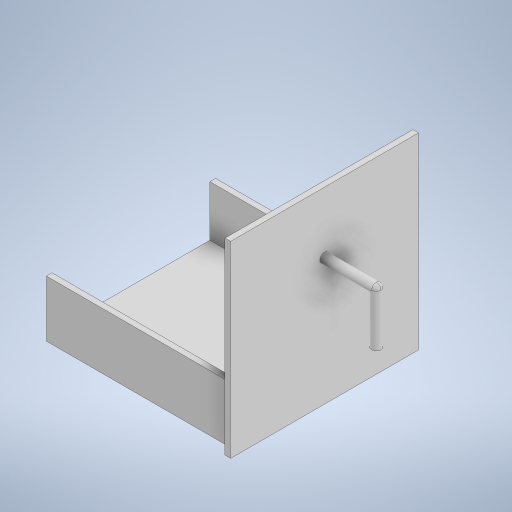
# Autodesk Inventor part: RS2_AshBucket
Saved by Autodesk Inventor 2024.3 (Build 283343000, 343)
## iProperties
Created: 2025-04-11
Part Number: RS2_AshBucket
Material: Generic
Document SubType Name: Modeling
Designer: ajclo
Density: 1 g/cm^3
Appearance: Default
Author: ajclo
Autodesk Inventor part; units mm, degrees
ref_plane "YZ Plane" through (0, 0, 0) normal (1, 0, 0) x (0, 1, 0)
ref_plane "XZ Plane" through (0, 0, 0) normal (0, 1, 0) x (-1, 0, 0)
ref_plane "XY Plane" through (0, 0, 0) normal (0, 0, 1) x (1, 0, 0)
sketch "Sketch1" plane through (0, 0, 0) normal (1, 0, 0) x (0, 1, 0)
  line L0 (0, 45) -> (30, 45)
  line L1 (30, 45) -> (30, -45)
  line L2 (30, -45) -> (0, -45)
  line L3 (0, -45) -> (0, 45)
  line L4 (30, 42) -> (3, 42)
  line L5 (3, 42) -> (3, -42)
  line L6 (3, -42) -> (30, -42)
  line L7 (30, -42) -> (30, 42)
  point P0 (0, 0)
  point P1 (30, -42)
  dimension "d0" = 45
  dimension "d1" = 90
  dimension "d2" = 30
  dimension "d3" = 0
  dimension "d4" = 3
  dimension "d5" = 3
  dimension "d6" = 3
  constraints: 16 end point, 4 parallel, 2 horizontal, 2 perpendicular, 1 point on line
  measures "d0" distance from line of L0 point (0, 0)
  measures "d1" distance of L0.end L1.end
  measures "d2" distance of L0.start L0.end
  measures "d3" distance from line of point (0, 0) L3
  measures "d4" distance between parallel lines of L2 L6
  measures "d5" distance between parallel lines of L3 L5
  measures "d6" distance between parallel lines of L0 L4
extrude "Extrusion1" add sketch "Sketch1" along normal blind 100 contours L0 L1 L4 L5 L6 L2 L3
sketch "Sketch2" plane through (100, 0, 0) normal (1, 0, 0) x (0, 0, -1)
  line L0 (-50, 0) -> (50, 0)
  line L1 (50, 0) -> (50, 100)
  line L2 (50, 100) -> (-50, 100)
  line L3 (-50, 100) -> (-50, 0)
  line L4 (-45, 0) -> (45, 0) projected
  point P0 (0, 0)
  point P1 (0, 0)
  dimension "d9" = 100
  dimension "d10" = 100
  constraints: 8 end point, 2 midpoint, 2 parallel, 1 horizontal, 1 perpendicular
  measures "d9" distance of L1.end L2.end
  measures "d10" distance of L0.end L1.end
extrude "Extrusion2" add sketch "Sketch2" along normal blind 3
sketch "Sketch4" plane through (0, 0, 0) normal (0, 0, 1) x (1, 0, 0)
  line L0 (103, 100) -> (103, 0) projected
  line L1 (103, 70) -> (133, 70)
  line L2 (133, 70) -> (133, 40)
  line L3 (133, 40) -> (128, 40)
  line L4 (128, 40) -> (128, 65)
  line L5 (128, 65) -> (103, 65)
  line L6 (100, 100) -> (103, 100) projected
  point P0 (0, 0)
  point P1 (115.5, 65)
  point P2 (118, 70)
  point P3 (128, 52.5)
  point P4 (101.5, 100)
  dimension "d13" = 5
  dimension "d14" = 5
  dimension "d15" = 30
  dimension "d16" = 30
  dimension "d17" = 30
  constraints: 10 end point, 4 midpoint, 4 perpendicular, 2 point on line, 1 horizontal
  measures "d13" vertical distance of point (115.5, 65) point (118, 70)
  measures "d14" distance from line of L2 point (128, 52.5)
  measures "d15" distance of L1.start L1.end
  measures "d16" distance of L1.end L2.end
  measures "d17" vertical distance of point (118, 70) point (101.5, 100)
extrude "Extrusion3" add sketch "Sketch4" along normal mid plane 5
fillet "Fillet1" radius 2.5 8 edges at (118, 70, 2.5) (115.5, 65, 2.5) (133, 55, 2.5) (128, 52.5, 2.5) (133, 55, -2.5) (133, 70, 0) (118, 70, -2.5) (115.5, 65, -2.5)
equation "\"d5\" = d4"
equation "\"d6\" = d4"
equation "\"d10\" = d9"
equation "\"d14\" = d13"
equation "\"d16\" = d15"
body "Solid1"
